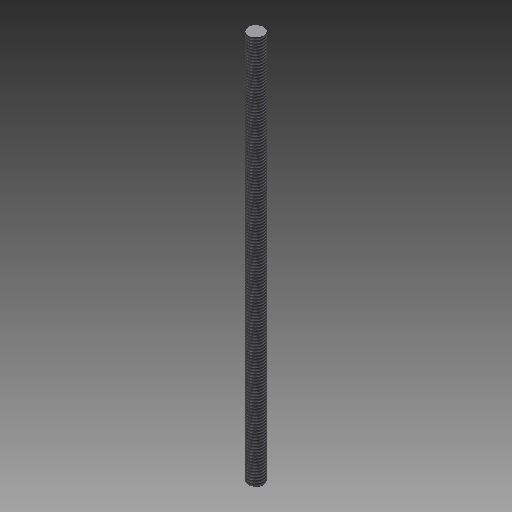
# Autodesk Inventor part: threaded_rod
Saved by Autodesk Inventor 2019 (Build 230136000, 136)
## iProperties
Created: 2014-07-14
Part Number: threaded_rod
Material: Generic
Document SubType Name: Modeling
Designer: cruiser
Density: 1 g/cm^3
Appearance: Default
Author: cruiser
Autodesk Inventor part; units mm, degrees
ref_plane "YZ Plane" through (0, 0, 0) normal (1, 0, 0) x (0, 1, 0)
ref_plane "XZ Plane" through (0, 0, 0) normal (0, 1, 0) x (-1, 0, 0)
ref_plane "XY Plane" through (0, 0, 0) normal (0, 0, 1) x (1, 0, 0)
sketch "Sketch1" plane through (0, 0, 0) normal (0, 1, 0) x (-1, 0, 0)
  circle A0 centre (0, 0) radius 3.9688
  dimension "d0" = 7.9375
  constraints: 1 centre point, 1 coincident
  measures "d0" diameter of A0
extrude "Extrusion1" add sketch "Sketch1" along normal blind 203.2
thread "Thread1" size "5/16-18 UNC" class "2A" standard "ANSI Unified Screw Threads" full length
equation "\"d1\" = threaded_rod_z"
equation "\"wood_thickness\" = 6.72"
equation "\"m3_diameter\" = 3.15"
equation "\"m5_diameter\" = 5.25"
equation "\"stepper_screw_space\" = 35"
equation "\"stepper_shaft_diameter\" = 5"
equation "\"stepper_body_diameter\" = 28"
equation "\"laser_body_diameter\" = 12"
equation "\"thick_acrylic\" = 5.88"
equation "\"carrier_y\" = 181"
equation "\"reservoir_x\" = 151"
equation "\"reservoir_y\" = 151"
equation "\"thin_acrylic\" = 3.15"
equation "\"linear_bearing_spacing\" = 207"
equation "\"linear_bearing_z\" = 304.8"
equation "\"threaded_rod_z\" = 203.2"
equation "\"motor_spacing\" = 287"
equation "\"tray_boarder\" = 15"
equation "\"tray_x\" = 151"
equation "\"tray_y\" = 181"
equation "\"brass_insert_drill\" = 4"
equation "\"brass_keep_out\" = 8"
equation "\"tape_keep_out\" = 2"
equation "\"tape_thickness\" = 2"
equation "\"crane_x\" = 244.56"
equation "\"z_min_from_center\" = 72.28"
equation "\"printer_z\" = 289"
equation "\"carrier_z\" = 233.04"
equation "\"carrier_z2\" = 283.04"
equation "\"window_z\" = 185"
equation "\"window_slot\" = 25"
equation "\"frame_tilt\" = 0"
equation "\"lcd_x\" = 72"
equation "\"lcd_y\" = 25"
equation "\"clear_acrylic\" = 3.15"
equation "\"laser_diameter\" = 12"
equation "\"laser_y_offset\" = 19.4"
equation "\"subframe_y_offset\" = 27.5"
equation "\"laser_y\" = 33"
equation "\"laser_z\" = 33"
equation "\"frame_top_z\" = 295"
equation "\"frame_bottom_z\" = 225"
equation "\"frame_y\" = 68.44"
equation "\"frame_border\" = 39.5"
equation "\"t_frame\" = 6.72"
equation "\"t_carrier\" = 6.72"
equation "\"t_tray\" = 3.15"
equation "\"tray_border\" = 15"
equation "\"t_wall\" = 5.88"
equation "\"galvo_frame_z\" = 65"
equation "\"galvo_frame_x\" = 66"
equation "\"t_galvo_frame\" = 6.72"
equation "\"galvo_frame_y_offset\" = 27.5"
equation "\"m4_diameter\" = 4.2"
equation "\"laser_z_offset\" = 55"
equation "\"window_y\" = 49.56"
equation "\"t_window\" = 3.15"
equation "\"laser_x\" = 62"
equation "\"drawer_y\" = 49.56"
equation "\"drawer_x\" = 181"
equation "\"drawer_z\" = 206.72"
equation "\"frame_foot_z\" = 49.5"
equation "\"drawer_z_from_bottom\" = 25"
equation "\"t_crane\" = 6.72"
equation "\"end_stop_offset_x\" = 83"
equation "\"end_stop_spacing\" = 19"
equation "\"thumb_nut_offset_y\" = 11.72"
equation "\"thumb_nut_diameter\" = 7"
equation "\"frame_foot_extension\" = 6"
equation "\"m5_brass_insert_drill\" = 6.7"
equation "\"m3_brass_insert_drill\" = 4"
equation "\"door_sensor\" = 35"
equation "\"protection_slot\" = 30.2"
equation "\"protection_slot_offset\" = 37.75"
equation "\"protection_slot_length\" = 20.6"
equation "\"m3_main_nut_width\" = 5.7"
equation "\"m3_main_extra\" = 1"
equation "\"m3_main_length\" = 14"
equation "\"m3_main_nut_thickness\" = 2.5"
equation "\"bed_t\" = 1.5875"
equation "\"al1_thickness\" = 1.5875"
equation "\"bed_fold_x\" = 15"
equation "\"bed_gap\" = 0.3"
equation "\"bed_y2\" = 45.96"
equation "\"m5_press_nut_drill\" = 6.35"
equation "\"asym_key\" = 0"
equation "\"small_round\" = 2"
equation "\"drawer_foot_mount\" = 18"
equation "\"inner_tray_x\" = 145"
equation "\"inner_tray_radius\" = 24"
equation "\"t_tape\" = 3"
equation "\"t_inner_tray\" = 5.88"
equation "\"inner_tray_y\" = 145"
equation "\"inner_tray_border\" = 5"
equation "\"bottom_clear_border\" = 5"
equation "\"t_bottom_clear\" = 3.15"
equation "\"laser_screw_spacing_y\" = 16"
body "Solid1"
